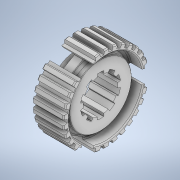
# Autodesk Inventor part: 74. Ступица муфты переключения третьей и четвертой передач
Saved by Autodesk Inventor 2021 (Build 250183000, 183)
## iProperties
Created: 2021-03-27
Part Number: 74. Ступица муфты переключения третьей и четвертой передач
Material: Типовые
Document SubType Name: Modeling
Designer: Данил
Density: 1 g/cm^3
Appearance: По умолчанию
Author: Данил
Autodesk Inventor part; units mm, degrees
ref_plane "YZ Plane" through (0, 0, 0) normal (1, 0, 0) x (0, 1, 0)
ref_plane "XZ Plane" through (0, 0, 0) normal (0, 1, 0) x (-1, 0, 0)
ref_plane "XY Plane" through (0, 0, 0) normal (0, 0, 1) x (1, 0, 0)
sketch "Эскиз1" plane through (0, 0, 0) normal (0, 0, 1) x (1, 0, 0)
  line L0 (-14.75, 0) -> (14.75, 0)
  line L1 (-14.75, -16.5) -> (-14.75, -24)
  line L2 (-14.75, -24) -> (-9.75, -24)
  line L3 (-4.75, -29) -> (-4.75, -34)
  line L4 (-5.75, -35) -> (-13.75, -35)
  line L5 (-14.75, -36) -> (-14.75, -40.5)
  line L6 (-14.75, -40.5) -> (14.75, -40.5)
  arc A0 (-5.75, -35) -> (-4.75, -34) centre (-5.75, -34) ccw
  arc A1 (-4.75, -29) -> (-9.75, -24) centre (-9.75, -29) ccw
  line L7 (-14.75, -16.5) -> (9.25, -16.5)
  line L8 (9.25, -16.5) -> (9.25, -29)
  line L9 (8.75, -29.5) -> (5.25, -29.5)
  line L10 (3.25, -31.5) -> (3.25, -34)
  line L11 (4.25, -35) -> (13.75, -35)
  line L12 (14.75, -36) -> (14.75, -40.5)
  arc A2 (5.25, -29.5) -> (3.25, -31.5) centre (5.25, -31.5) ccw
  arc A3 (3.25, -34) -> (4.25, -35) centre (4.25, -34) ccw
  line L13 (8.75, -29.5) -> (9.25, -29)
  line L14 (13.75, -35) -> (14.75, -36)
  line L15 (-13.75, -35) -> (-14.75, -36)
  point P0 (0, 0)
  point P1 (0, 0)
  point P2 (-14.75, -35)
  point P3 (9.25, -29.5)
  point P4 (14.75, -35)
  dimension "d0" = 29.5
  dimension "d2" = 70
  dimension "d3" = 81
  dimension "d4" = 10
  dimension "d5" = 1
  dimension "d6" = 5
  dimension "d7" = 48
  dimension "d8" = 33
  dimension "d9" = 11.5
  dimension "d10" = 70
  dimension "d11" = 59
  dimension "d12" = 5.5
  dimension "d13" = 2
  dimension "d14" = 1
  dimension "d15" = 0.5
  dimension "d16" = 45
  dimension "d17" = 1
  dimension "d18" = 45
  dimension "d19" = 1
  dimension "d20" = 45
  constraints: 32 end point, 8 perpendicular, 8 point on circle, 8 point on line, 8 tangent, 4 centre point, 2 vertical, 2 vertical alignment, 1 coincident, 1 horizontal, 1 midpoint
  measures "d0" distance of L0.start L0.end
  measures "d2" diameter of L4 L0
  measures "d3" diameter of L6 L0
  measures "d4" distance between parallel lines of L5 L3
  measures "d5" radius of A0
  measures "d6" radius of A1
  measures "d7" diameter of L2 L0
  measures "d8" diameter of L7 L0
  measures "d9" distance from line of L0.end L10
  measures "d10" diameter of L11 L0
  measures "d11" diameter of L9 L0
  measures "d12" distance from line of L0.end L8
  measures "d13" radius of A2
  measures "d14" radius of A3
  measures "d15" distance of L9.start point (9.25, -29.5)
  measures "d16" angle of L9 L13
  measures "d17" distance of L11.end point (14.75, -35)
  measures "d18" angle of L11 L14
  measures "d19" distance of L4.end point (-14.75, -35)
  measures "d20" angle of L4 L15
revolve "Вращение1" add sketch "Эскиз1" angle 360 about axis through (-14.75, 0, 0) along (1, 0, 0)
sketch "Эскиз2" plane through (-14.75, 0, 0) normal (-1, 0, 0) x (0, 0, 1)
  circle A0 centre (0, 0) radius 16.5 projected
  circle A1 centre (0, 0) radius 19
  circle A2 centre (0, 0) radius 16.5 projected
  line L0 (-3, 16.225) -> (-3, 18.7617)
  line L1 (3, 16.225) -> (3, 18.7617)
  line L2 (-3, 16.225) -> (3, 16.225) construction
  line L3 (-11.9639, 11.3629) -> (-13.4549, 13.4151)
  line L4 (-7.1098, 14.8896) -> (-8.6008, 16.9419)
  line L5 (-16.3579, 2.1606) -> (-18.7705, 2.9445)
  line L6 (-14.5038, 7.867) -> (-16.9164, 8.6508)
  line L7 (-14.5038, -7.867) -> (-16.9164, -8.6508)
  line L8 (-16.3579, -2.1606) -> (-18.7705, -2.9445)
  line L9 (-7.1098, -14.8896) -> (-8.6008, -16.9419)
  line L10 (-11.9639, -11.3629) -> (-13.4549, -13.4151)
  line L11 (3, -16.225) -> (3, -18.7617)
  line L12 (-3, -16.225) -> (-3, -18.7617)
  line L13 (11.9639, -11.3629) -> (13.4549, -13.4151)
  line L14 (7.1098, -14.8896) -> (8.6008, -16.9419)
  line L15 (16.3579, -2.1606) -> (18.7705, -2.9445)
  line L16 (14.5038, -7.867) -> (16.9164, -8.6508)
  line L17 (14.5038, 7.867) -> (16.9164, 8.6508)
  line L18 (16.3579, 2.1606) -> (18.7705, 2.9445)
  line L19 (7.1098, 14.8896) -> (8.6008, 16.9419)
  line L20 (11.9639, 11.3629) -> (13.4549, 13.4151)
  point P0 (0, 0)
  dimension "d22" = 38
  dimension "d23" = 6
  dimension "d26" = 360
  constraints: 42 end point, 4 point on circle, 1 centre point, 1 coincident, 1 horizontal, 1 parallel, 1 vertical, 61 other
  measures "d22" diameter of A1
  measures "d23" distance of L0.start L1.start
extrude "Выдавливание1" cut sketch "Эскиз2" against normal up to surface (24 mm away) contours A0 L17 A1 L18 | L15 A1 L16 A0 | A0 L19 A1 L20 | L13 A1 L14 A0 | A0 L0 A1 L1 | L11 A1 L12 A0 | A0 L3 A1 L4 | L9 A1 L10 A0 | A0 L5 A1 L6 | L7 A1 L8 A0
fillet "Сопряжение1" radius 0.2 20 edges at (-2.75, -2.9445, -18.7705) (-2.75, 2.9445, -18.7705) (-2.75, 8.6508, -16.9164) (-2.75, 13.4151, -13.4549) (-2.75, 16.9419, -8.6008) (-2.75, 18.7617, -3) (-2.75, 18.7617, 3) (-2.75, 16.9419, 8.6008) (-2.75, 13.4151, 13.4549) (-2.75, 8.6508, 16.9164) (-2.75, 2.9445, 18.7705) (-2.75, -2.9445, 18.7705) (-2.75, -8.6508, 16.9164) (-2.75, -13.4151, 13.4549) (-2.75, -16.9419, 8.6008) (-2.75, -18.7617, 3) (-2.75, -18.7617, -3) (-2.75, -16.9419, -8.6008) (-2.75, -13.4151, -13.4549) (-2.75, -8.6508, -16.9164)
sketch "Эскиз3" plane through (-14.75, 0, 0) normal (-1, 0, 0) x (0, 0, 1)
  circle A0 centre (0, 0) radius 40.5 projected
  circle A1 centre (0, 0) radius 39 construction
  line L0 (-2.3652, 36.9602) -> (-1.7957, 40.4602)
  circle A2 centre (0, 0) radius 40.5 construction
  line L1 (2.3652, 36.9602) -> (1.7957, 40.4602)
  line L2 (-2.042, 38.9465) -> (2.042, 38.9465) construction
  circle A3 centre (0, 0) radius 37.0358
  line L3 (-9.998, 35.6607) -> (-10.1686, 39.2027)
  line L4 (-5.3709, 36.6443) -> (-6.6557, 39.9494)
  line L5 (-17.1938, 32.8028) -> (-18.0971, 36.2318)
  line L6 (-12.8723, 34.7268) -> (-14.8162, 37.6926)
  line L7 (-23.6382, 28.5112) -> (-25.2346, 31.6775)
  line L8 (-19.8111, 31.2917) -> (-22.3292, 33.7884)
  line L9 (-29.0494, 22.9735) -> (-31.2693, 25.7387)
  line L10 (-25.8841, 26.4889) -> (-28.8662, 28.4076)
  line L11 (-33.1911, 16.4317) -> (-35.9374, 18.675)
  line L12 (-30.8258, 20.5284) -> (-34.1417, 21.7852)
  line L13 (-35.8821, 9.1718) -> (-39.0348, 10.7951)
  line L14 (-34.4203, 13.6708) -> (-37.925, 14.2107)
  line L15 (-37.0049, 1.5111) -> (-40.4262, 2.4434)
  line L16 (-36.5105, 6.2157) -> (-40.0508, 6.0151)
  line L17 (-36.5105, -6.2157) -> (-40.0508, -6.0151)
  line L18 (-37.0049, -1.5111) -> (-40.4262, -2.4434)
  line L19 (-34.4203, -13.6708) -> (-37.925, -14.2107)
  line L20 (-35.8821, -9.1718) -> (-39.0348, -10.7951)
  line L21 (-30.8258, -20.5284) -> (-34.1417, -21.7852)
  line L22 (-33.1911, -16.4317) -> (-35.9374, -18.675)
  line L23 (-25.8841, -26.4889) -> (-28.8662, -28.4076)
  line L24 (-29.0494, -22.9735) -> (-31.2693, -25.7387)
  line L25 (-19.8111, -31.2917) -> (-22.3292, -33.7884)
  line L26 (-23.6382, -28.5112) -> (-25.2346, -31.6775)
  line L27 (-12.8723, -34.7268) -> (-14.8162, -37.6926)
  line L28 (-17.1938, -32.8028) -> (-18.0971, -36.2318)
  line L29 (-5.3709, -36.6443) -> (-6.6557, -39.9494)
  line L30 (-9.998, -35.6607) -> (-10.1686, -39.2027)
  line L31 (2.3652, -36.9602) -> (1.7957, -40.4602)
  line L32 (-2.3652, -36.9602) -> (-1.7957, -40.4602)
  line L33 (9.998, -35.6607) -> (10.1686, -39.2027)
  line L34 (5.3709, -36.6443) -> (6.6557, -39.9494)
  line L35 (17.1938, -32.8028) -> (18.0971, -36.2318)
  line L36 (12.8723, -34.7268) -> (14.8162, -37.6926)
  line L37 (23.6382, -28.5112) -> (25.2346, -31.6775)
  line L38 (19.8111, -31.2917) -> (22.3292, -33.7884)
  line L39 (29.0494, -22.9735) -> (31.2693, -25.7387)
  line L40 (25.8841, -26.4889) -> (28.8662, -28.4076)
  line L41 (33.1911, -16.4317) -> (35.9374, -18.675)
  line L42 (30.8258, -20.5284) -> (34.1417, -21.7852)
  line L43 (35.8821, -9.1718) -> (39.0348, -10.7951)
  line L44 (34.4203, -13.6708) -> (37.925, -14.2107)
  line L45 (37.0049, -1.5111) -> (40.4262, -2.4434)
  line L46 (36.5105, -6.2157) -> (40.0508, -6.0151)
  line L47 (36.5105, 6.2157) -> (40.0508, 6.0151)
  line L48 (37.0049, 1.5111) -> (40.4262, 2.4434)
  line L49 (34.4203, 13.6708) -> (37.925, 14.2107)
  line L50 (35.8821, 9.1718) -> (39.0348, 10.7951)
  line L51 (30.8258, 20.5284) -> (34.1417, 21.7852)
  line L52 (33.1911, 16.4317) -> (35.9374, 18.675)
  line L53 (25.8841, 26.4889) -> (28.8662, 28.4076)
  line L54 (29.0494, 22.9735) -> (31.2693, 25.7387)
  line L55 (19.8111, 31.2917) -> (22.3292, 33.7884)
  line L56 (23.6382, 28.5112) -> (25.2346, 31.6775)
  line L57 (12.8723, 34.7268) -> (14.8162, 37.6926)
  line L58 (17.1938, 32.8028) -> (18.0971, 36.2318)
  line L59 (5.3709, 36.6443) -> (6.6557, 39.9494)
  line L60 (9.998, 35.6607) -> (10.1686, 39.2027)
  point P0 (0, 0)
  point P1 (0, 38.9465)
  point P2 (-10.0948, 37.6709)
  point P3 (-6.1001, 38.52)
  point P4 (-17.7064, 34.7488)
  point P5 (-13.9755, 36.41)
  point P6 (-24.5442, 30.3081)
  point P7 (-21.2402, 32.7086)
  point P8 (-30.3093, 24.5428)
  point P9 (-27.5765, 27.5778)
  point P10 (-34.7497, 17.7048)
  point P11 (-32.7077, 21.2417)
  point P12 (-37.6713, 10.0931)
  point P13 (-36.4093, 13.9772)
  point P14 (-38.9466, 2.0402)
  point P15 (-38.5197, 6.1018)
  point P16 (-38.5197, -6.1018)
  point P17 (-38.9466, -2.0402)
  point P18 (-36.4093, -13.9772)
  point P19 (-37.6713, -10.0931)
  point P20 (-32.7077, -21.2417)
  point P21 (-34.7497, -17.7048)
  point P22 (-27.5765, -27.5778)
  point P23 (-30.3093, -24.5428)
  point P24 (-21.2402, -32.7086)
  point P25 (-24.5442, -30.3081)
  point P26 (-13.9755, -36.41)
  point P27 (-17.7064, -34.7488)
  point P28 (-6.1001, -38.52)
  point P29 (-10.0948, -37.6709)
  point P30 (2.042, -38.9465)
  point P31 (-2.042, -38.9465)
  point P32 (10.0948, -37.6709)
  point P33 (6.1001, -38.52)
  point P34 (17.7064, -34.7488)
  point P35 (13.9755, -36.41)
  point P36 (24.5442, -30.3081)
  point P37 (21.2402, -32.7086)
  point P38 (30.3093, -24.5428)
  point P39 (27.5765, -27.5778)
  point P40 (34.7497, -17.7048)
  point P41 (32.7077, -21.2417)
  point P42 (37.6713, -10.0931)
  point P43 (36.4093, -13.9772)
  point P44 (38.9466, -2.0402)
  point P45 (38.5197, -6.1018)
  point P46 (38.5197, 6.1018)
  point P47 (38.9466, 2.0402)
  point P48 (36.4093, 13.9772)
  point P49 (37.6713, 10.0931)
  point P50 (32.7077, 21.2417)
  point P51 (34.7497, 17.7048)
  point P52 (27.5765, 27.5778)
  point P53 (30.3093, 24.5428)
  point P54 (21.2402, 32.7086)
  point P55 (24.5442, 30.3081)
  point P56 (13.9755, 36.41)
  point P57 (17.7064, 34.7488)
  point P58 (6.1001, 38.52)
  point P59 (10.0948, 37.6709)
  dimension "d31" = 78
  dimension "d32" = 4.084
  dimension "d33" = 3.5
  dimension "d34" = 74.0716
  dimension "d37" = 360
  constraints: 122 end point, 60 point on line, 4 point on circle, 2 centre point, 2 coincident, 1 equal length, 1 midpoint, 1 vertical alignment, 245 other
  measures "d31" diameter of A1
  measures "d32" distance of L2.start L2.end
  measures "d33" vertical distance of L1.start L1.end
  measures "d34" diameter of A3
chamfer "Фаска1" distance 1 angle 45 1 edges at (-14.75, 40.5, 0) measured on face at (-14.75, -2.1169, 37.2776)
chamfer "Фаска2" distance 1 angle 45 1 edges at (14.75, 40.5, 0) measured on face at (14.75, -2.1169, 37.2776)
extrude "Выдавливание2" cut sketch "Эскиз3" against normal through all contours L59 A3 L1 A0
pattern_circular "Круговой массив1" count 30 over 360 about axis through (0, 0, 0) along (-1, 0, 0) of "Выдавливание2"
sketch "Эскиз4" plane through (-14.75, 0, 0) normal (-1, 0, 0) x (0, 0, 1)
  line L0 (-47.5, 6.5) -> (-32.5, 6.5)
  line L1 (-32.5, 6.5) -> (-32.5, -6.5)
  line L2 (-32.5, -6.5) -> (-47.5, -6.5)
  line L3 (-47.5, -6.5) -> (-47.5, 6.5)
  point P0 (0, 0)
  point P1 (-47.5, 0)
  dimension "d50" = 13
  dimension "d51" = 32.5
  dimension "d52" = 15
  constraints: 8 end point, 2 parallel, 1 horizontal, 1 horizontal alignment, 1 midpoint, 1 perpendicular
  measures "d50" distance of L2.end L0.start
  measures "d51" distance from line of L1 point (0, 0)
  measures "d52" distance of L0.start L0.end
extrude "Выдавливание3" cut sketch "Эскиз4" against normal through all
pattern_circular "Круговой массив2" count 3 over 360 about axis through (-12.25, 0, 0) along (-1, 0, 0) of "Выдавливание3"
equation "\"d19\" = d17"
equation "\"d20\" = d18"
